003 (Autodesk Fusion 360 design; units mm, degrees)
Autodesk Fusion 360 part; units mm, degrees
sketch "Esquisse1" plane through (0, 0, 0) normal (1, 0, 0) x (0, 1, 0)
  line L0 (13.5, 3) -> (13.5, 0)
  line L1 (13.5, 0) -> (14.5, 0)
  line L2 (14.5, 0) -> (14.5, 5)
  line L3 (14.5, 5) -> (9, 5)
  line L4 (9, 15) -> (8.5, 15)
  line L5 (8.5, 15) -> (8.5, 47)
  line L6 (8.5, 47) -> (0, 47)
  line L7 (0, 47) -> (0, 3)
  line L8 (0, 3) -> (13.5, 3)
  line L9 (9, 15) -> (9, 5)
  dimension "d33" = 3
  dimension "d34" = 13.5
  dimension "d35" = 1
  dimension "d36" = 5
  dimension "d40" = 32
  dimension "d41" = 8.5
  dimension "d43" = 9
  dimension "d44" = 10
  constraint vertical L0
  constraint perpendicular L0 L1
  constraint perpendicular L1 L2
  constraint perpendicular L2 L3
  constraint perpendicular L4 L5
  constraint perpendicular L5 L6
  constraint perpendicular L6 L7
  constraint horizontal L8
  constraint coincident origin L7
  constraint coincident origin L1
  constraint vertical L9
  measures "d33" distance of L0.start L0.end
  measures "d34" distance of origin L0
  measures "d35" distance of L0.end L1.end
  measures "d36" distance of L1.end L2.end
  measures "d40" distance of L4.end L5.end
  measures "d41" distance of L5.end L6.end
  measures "d43" distance of L7 L9
  measures "d44" distance of L3.end L4.start
revolve "Révolution1" add sketch "Esquisse1" angle 360 about axis through (0, 0, 47) along (0, 0, -1)
sketch "Esquisse1 (2)" plane through (0, 0, 5) normal (0, 0, 1) x (-1, 0, 0)
sketch "Esquisse2" plane through (0, 0, 5) normal (0, 0, 1) x (1, 0, 0)
  circle A0 centre (0, 0) radius 11.75 construction
  circle A1 centre (0, -11.75) radius 1.5
  dimension "d57" = 23.5
  dimension "d58" = 3
  constraint coincident A0.centre origin
  constraint coincident A0 A1.centre
  measures "d57" diameter of A0
  measures "d58" diameter of A1
extrude "Extrusion1" cut sketch "Esquisse2" against normal blind 4
pattern_circular "Réseau C1" count 3 over 360 about axis through (0, 0, 47) along (0, 0, -1) of "Extrusion1"
equation "d41 = ( 17 / 2 ) * 1 mm"
